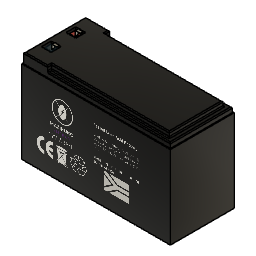
MMC - Lead Acid Battery (Autodesk Fusion 360 design; units mm, degrees)
Autodesk Fusion 360 part; units mm, degrees
sketch "Sketch1" plane through (0, 0, 0) normal (0, 0, 1) x (1, 0, 0)
  line L0 (0, 0) -> (151, 0)
  line L1 (151, 0) -> (151, -65)
  line L2 (151, -65) -> (0, -65)
  line L3 (0, -65) -> (0, 0)
  dimension "d1" = 151
  dimension "d2" = 65
  constraint horizontal L0
  constraint vertical L1
  constraint horizontal L2
  constraint vertical L3
  constraint coincident L0.start L3.end
  measures "d1" distance of L0.start L0.end
  measures "d2" distance of L0.start L2.end
extrude "Extrude1" add sketch "Sketch1" along normal blind 84 makes body 1
sketch "Sketch2" plane through (0, 0, 84) normal (0, 0, 1) x (-1, 0, 0)
  line L0 (0, 65) -> (-151, 65)
  line L1 (-151, 65) -> (-151, 0)
  line L2 (-151, 0) -> (0, 0)
  line L3 (0, 0) -> (0, 65)
  line L4 (-1, 1) -> (-150, 1)
  line L5 (-150, 1) -> (-150, 64)
  line L6 (-150, 64) -> (-1, 64)
  line L7 (-1, 64) -> (-1, 1)
  dimension "d5" = 1
  dimension "d6" = 1
  dimension "d7" = 1
  dimension "d8" = 1
  constraint horizontal L4
  constraint vertical L5
  constraint horizontal L6
  constraint vertical L7
  measures "d5" distance of L2 L4
  measures "d6" distance of L1 L5
  measures "d7" distance of L0 L6
  measures "d8" distance of L3 L7
extrude "Extrude2" add sketch "Sketch2" along normal blind 5 separate body contours L4 L5 L6 L7 makes body 2
sketch "Sketch3" plane through (0, 0, 89) normal (0, 0, 1) x (-1, 0, 0)
  line L0 (-1, 64) -> (-150, 64)
  line L1 (-150, 64) -> (-150, 1)
  line L2 (-150, 1) -> (-1, 1)
  line L3 (-1, 1) -> (-1, 64)
  line L4 (-1, 1) -> (-25.3263, 1)
  line L5 (-25.3263, 64) -> (-1, 64)
  line L6 (-1, 64) -> (-1, 1)
  line L7 (-25.3263, 5.5031) -> (-145, 5.5031)
  line L8 (-145, 5.5031) -> (-145, 60)
  line L9 (-145, 60) -> (-25.3263, 60)
  line L10 (-25.3263, 1) -> (-25.3263, 5.5031)
  line L11 (-25.3263, 60) -> (-25.3263, 64)
  constraint horizontal L4
  constraint vertical L10
  constraint horizontal L5
  constraint vertical L6
  constraint coincident L0 L5.start
  constraint coincident L2.end L3.start
  constraint horizontal L7
  constraint vertical L8
  constraint horizontal L9
  constraint collinear L10 L11
extrude "Extrude3" add sketch "Sketch3" along normal blind 5 contours L0 L2 L3 L4 L5 L6 L7 L8 L9 L10 L11 bodies 2
sketch "Sketch4" plane through (0, 0, 94) normal (0, 0, 1) x (-1, 0, 0)
  line L0 (-25.3263, 60) -> (-145, 60)
  line L1 (-145, 60) -> (-145, 5.5031)
  line L2 (-145, 5.5031) -> (-25.3263, 5.5031)
  line L3 (-25.3263, 5.5031) -> (-25.3263, 1)
  line L4 (-25.3263, 1) -> (-1, 1)
  line L5 (-1, 1) -> (-1, 64)
  line L6 (-1, 64) -> (-25.3263, 64)
  line L7 (-25.3263, 64) -> (-25.3263, 60)
  line L8 (-5, 15) -> (-15, 15)
  line L9 (-15, 15) -> (-15, 25)
  line L10 (-15, 25) -> (-5, 25)
  line L11 (-5, 25) -> (-5, 15)
  line L12 (-15, 50) -> (-5, 50)
  line L13 (-5, 50) -> (-5, 40)
  line L14 (-5, 40) -> (-15, 40)
  line L15 (-15, 40) -> (-15, 50)
  constraint horizontal L8
  constraint vertical L9
  constraint horizontal L10
  constraint vertical L11
  constraint horizontal L12
  constraint vertical L13
  constraint horizontal L14
  constraint vertical L15
extrude "Extrude4" cut sketch "Sketch4" against normal blind 1 contours L8 L9 L10 L11 | L12 L13 L14 L15 bodies 2
fillet "Fillet1" radius 2 8 edges at (10, -15, 93) (5, -20, 93) (15, -20, 93) (10, -25, 93) (15, -45, 93) (10, -50, 93) (5, -45, 93) (10, -40, 93) on bodies 2
sketch "Sketch5" plane through (0, 0, 93) normal (0, 0, 1) x (-1, 0, 0)
  line L0 (-13.2679, 41.7321) -> (-6.7321, 41.7321)
  line L1 (-6.7321, 41.7321) -> (-6.7321, 48.2679)
  line L2 (-6.7321, 48.2679) -> (-13.2679, 48.2679)
  line L3 (-13.2679, 48.2679) -> (-13.2679, 41.7321)
sketch "Sketch6" plane through (0, 0, 93) normal (0, 0, 1) x (-1, 0, 0)
  line L0 (-12, 46.5) -> (-11.9, 46.5)
  line L1 (-11.9, 46.5) -> (-11.9, 43.4435)
  line L2 (-11.9, 43.4435) -> (-12, 43.4435)
  line L3 (-12, 43.4435) -> (-12, 46.5)
  dimension "d17" = 0.1
  constraint horizontal L0
  constraint vertical L1
  constraint horizontal L2
  constraint vertical L3
  measures "d17" distance of L0.start L0.end
extrude "Extrude5" add sketch "Sketch6" along normal blind 5 separate body makes body 3
sketch "Sketch7" plane through (12, 0, 0) normal (1, 0, 0) x (0, 1, 0)
  line L0 (-46.5, 93) -> (-43.4435, 93)
  line L1 (-43.4435, 93) -> (-43.4435, 98)
  line L2 (-43.4435, 98) -> (-46.5, 98)
  line L3 (-46.5, 98) -> (-46.5, 93)
  line L4 (-46.5, 98) -> (-43.4435, 98)
  line L5 (-43.4435, 98) -> (-43.4435, 97.9)
  line L6 (-43.4435, 97.9) -> (-46.5, 97.9)
  line L7 (-46.5, 97.9) -> (-46.5, 98)
  dimension "d20" = 0.1
  constraint horizontal L4
  constraint vertical L5
  constraint horizontal L6
  constraint vertical L7
  constraint coincident L1 L5.end
  constraint coincident L2.end L3.start
  measures "d20" distance of L4 L6
extrude "Extrude6" add sketch "Sketch7" along normal blind 5 contours L1 L2 L3 L4 L5 L6 L7 bodies 3
fillet "Fillet2" radius 0.3 1 edges at (11.9, -44.9718, 98) on bodies 3
pattern_linear "R-Pattern1" count 2 spacing 24 along (0, 1, 0) of bodies 3 makes body 4
fillet "Fillet3" radius 1 8 edges at (1, -32.5, 94) (13.1631, -1, 94) (13.1631, -64, 94) (25.3263, -62, 94) (85.1631, -60, 94) (145, -32.7515, 94) (85.1631, -5.5031, 94) (25.3263, -3.2515, 94) on bodies 2
fillet "Fillet4" radius 1 8 edges at (87.6631, -64, 89) (25.3263, -62, 89) (85.1631, -60, 89) (145, -32.7515, 89) (150, -32.5, 89) (85.1631, -5.5031, 89) (87.6631, -1, 89) (25.3263, -3.2515, 89) on bodies 2
